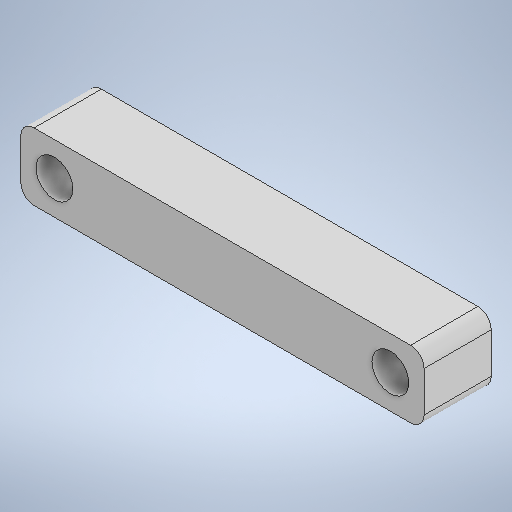
# Autodesk Inventor part: element_posredni_2
Saved by Autodesk Inventor 2025.2 (Build 292293000, 293)
## iProperties
Created: 2025-11-26
Part Number: element_posredni_2
Material: Ogólny
Document SubType Name: Modeling
Designer: juras
Density: 1 g/cm^3
Appearance: Domyślna
Author: juras
Autodesk Inventor part; units mm, degrees
ref_plane "YZ Plane" through (0, 0, 0) normal (1, 0, 0) x (0, 1, 0)
ref_plane "XZ Plane" through (0, 0, 0) normal (0, 1, 0) x (-1, 0, 0)
ref_plane "XY Plane" through (0, 0, 0) normal (0, 0, 1) x (1, 0, 0)
sketch "Szkic1" plane through (0, 0, 0) normal (0, 1, 0) x (-1, 0, 0)
  line L0 (-30, -5) -> (30, -5)
  line L1 (30, -5) -> (30, 5)
  line L2 (30, 5) -> (-30, 5)
  line L3 (-30, 5) -> (-30, -5)
  line L4 (-30, -5) -> (30, 5) construction
  line L5 (30, -5) -> (-30, 5) construction
  point P0 (0, 0)
  dimension "d0" = 60
  dimension "d1" = 10
  constraints: 12 end point, 2 midpoint, 2 parallel, 1 horizontal, 1 perpendicular
  measures "d0" distance of L2.end L1.end
  measures "d1" distance of L1.end L0.end
extrude "Wyciągnięcie proste1" add sketch "Szkic1" along normal mid plane 10
sketch "Szkic2" plane through (-30, 5, 5) normal (0, 0, 1) x (1, 0, 0)
  circle A0 centre (5, -5) radius 2.75
  line L0 (0, -10) -> (0, 0) projected
  line L1 (0, 0) -> (60, 0) projected
  point P0 (30, -5)
  dimension "d4" = 5
  dimension "d5" = 5
  dimension "d6" = 5.5
  constraints: 1 centre point
  measures "d4" distance from line of A0.centre L0
  measures "d5" distance from line of A0.centre L1
  measures "d6" diameter of A0
hole "Otwór1" at (-25, 0, 5) direction (0, 0, -1) diameter 5.5 end through all
mirror "Odbij1" about plane through (0, 0, 0) normal (1, 0, 0) of "Otwór1"
fillet "Zaokrąglenie1" radius 2 4 edges at (30, -5, 0) (30, 5, 0) (-30, -5, 0) (-30, 5, 0)
